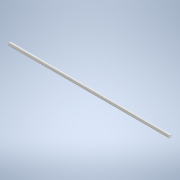
# Autodesk Inventor part: IntakeHexShaft
Saved by Autodesk Inventor 2021 (Build 250183000, 183)
## iProperties
Created: 2021-05-21
Part Number: IntakeHexShaft
Material: Generic
Document SubType Name: Modeling
Designer: sami8
Density: 1 g/cm^3
Appearance: Default
Author: sami8
Autodesk Inventor part; units mm, degrees
ref_plane "YZ Plane" through (0, 0, 0) normal (1, 0, 0) x (0, 1, 0)
ref_plane "XZ Plane" through (0, 0, 0) normal (0, 1, 0) x (-1, 0, 0)
ref_plane "XY Plane" through (0, 0, 0) normal (0, 0, 1) x (1, 0, 0)
sketch "Sketch1" plane through (0, 0, 0) normal (1, 0, 0) x (0, 1, 0)
  line L0 (2.5, -1.4434) -> (0, -2.8868)
  line L1 (0, -2.8868) -> (-2.5, -1.4434)
  line L2 (-2.5, -1.4434) -> (-2.5, 1.4434)
  line L3 (-2.5, 1.4434) -> (0, 2.8868)
  line L4 (0, 2.8868) -> (2.5, 1.4434)
  line L5 (2.5, 1.4434) -> (2.5, -1.4434)
  point P0 (0, 0)
  point P1 (0, 0)
  dimension "d0" = 5
  constraints: 12 end point, 1 coincident, 1 vertical, 13 other
  measures "d0" distance between parallel lines of L5 L2
extrude "Extrusion1" add sketch "Sketch1" along normal blind 289
body "Solid1"
